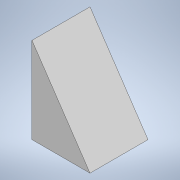
# Autodesk Inventor part: N1
Saved by Autodesk Inventor 2022 (Build 260153000, 153)
## iProperties
Created: 2023-03-30
Part Number: N1
Material: Типовые
Document SubType Name: Modeling
Designer: Hp
Density: 1 g/cm^3
Appearance: По умолчанию
Author: Hp
Autodesk Inventor part; units mm, degrees
ref_plane "YZ Plane" through (0, 0, 0) normal (1, 0, 0) x (0, 1, 0)
ref_plane "XZ Plane" through (0, 0, 0) normal (0, 1, 0) x (-1, 0, 0)
ref_plane "XY Plane" through (0, 0, 0) normal (0, 0, 1) x (1, 0, 0)
sketch "Эскиз1" plane through (0, 0, 0) normal (0, 0, 1) x (1, 0, 0)
  line L0 (0, 0) -> (10, 0)
  line L1 (10, 0) -> (0, 14.8256)
  line L2 (0, 0) -> (0, 14.8256)
  dimension "d0" = 10
  dimension "d1" = 56
  constraints: 6 end point, 1 horizontal, 1 vertical
  measures "d0" distance of L0.start L0.end
  measures "d1" angle of L1 L0
extrude "Выдавливание1" add sketch "Эскиз1" along normal blind 10
